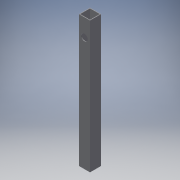
# Autodesk Inventor part: CounterWeight
Saved by Autodesk Inventor 2019.3 (Build 233278000, 278)
## iProperties
Created: 2019-07-02
Part Number: CounterWeight
Material: Generic
Document SubType Name: Modeling
Designer: mark
Density: 1 g/cm^3
Appearance: Default
Author: mark
Autodesk Inventor part; units mm, degrees
ref_plane "YZ Plane" through (0, 0, 0) normal (1, 0, 0) x (0, 1, 0)
ref_plane "XZ Plane" through (0, 0, 0) normal (0, 1, 0) x (-1, 0, 0)
ref_plane "XY Plane" through (0, 0, 0) normal (0, 0, 1) x (1, 0, 0)
sketch "Sketch1" plane through (0, 0, 0) normal (0, 0, 1) x (1, 0, 0)
  line L0 (0, 0) -> (25.4, 0) projected
  line L1 (25.4, 0) -> (25.4, 500) projected
  line L2 (0, 500) -> (25.4, 500) projected
  line L3 (0, 0) -> (0, 500) projected
  line L4 (23.8125, 0) -> (23.8125, 500) projected
  line L5 (1.5875, 0) -> (1.5875, 500) projected
  line L6 (25.4, 50) -> (0, 50)
  line L7 (0, 50) -> (0, -250)
  line L8 (0, -250) -> (25.4, -250)
  line L9 (25.4, -250) -> (25.4, 50)
  dimension "d0" = 50
  dimension "d1" = 300
  constraints: 8 end point, 2 collinear
  measures "d0" distance between parallel lines of L6 L0
  measures "d1" distance between parallel lines of L6 L8
extrude "Extrusion1" add sketch "Sketch1" along normal blind 25.4 contours L3 L6 L5 L0 | L0 L9 L8 L7 | L5 L6 L4 L0 | L4 L6 L1 L0
sketch "Sketch2" plane through (0, 50, 0) normal (0, 1, 0) x (1, 0, 0)
  line L0 (23.8125, -1.5875) -> (1.5875, -1.5875)
  line L1 (1.5875, -1.5875) -> (1.5875, -23.8125)
  line L2 (1.5875, -23.8125) -> (23.8125, -23.8125)
  line L3 (23.8125, -23.8125) -> (23.8125, -1.5875)
  line L4 (23.8125, 23.8125) -> (23.8125, 1.5875) projected
  line L5 (1.5875, 1.5875) -> (1.5875, 23.8125) projected
  line L6 (25.4, -25.4) -> (0, -25.4) projected
  point P0 (0, 0)
  dimension "d4" = 22.225
  dimension "d5" = 1.5875
  constraints: 8 end point, 2 collinear
  measures "d4" distance between parallel lines of L2 L0
  measures "d5" distance between parallel lines of L2 L6
extrude "Extrusion2" cut sketch "Sketch2" against normal up to next
sketch "Sketch3" plane through (0, 0, 25.4) normal (0, 0, 1) x (1, 0, 0)
  circle A0 centre (12.7, 10) radius 7.5
  line L0 (25.4, -250) -> (25.4, 50) projected
  line L1 (0, 0) -> (25.4, 0) projected
  line L2 (0, 0) -> (25.4, 0) projected
  line L3 (23.8125, 15.05) -> (1.5875, 15.05)
  dimension "d8" = 15
  dimension "d9" = 12.7
  dimension "d10" = 10
  constraints: 2 end point, 1 centre point, 1 horizontal, 2 other
  measures "d8" diameter of A0
  measures "d9" distance from line of L0 A0.centre
  measures "d10" distance from line of L1 A0.centre
extrude "Extrusion3" cut sketch "Sketch3" against normal up to next
sketch "Sketch4" plane through (1.5875, 50, 1.5875) normal (0, 0, 1) x (1, 0, 0)
  circle A0 centre (11.1125, -40) radius 7.5 projected
  circle A1 centre (11.1125, -40) radius 4.5
  point P0 (-1.5875, -50)
  dimension "d13" = 9
  constraints: 1 centre point, 1 coincident
  measures "d13" diameter of A1
extrude "Extrusion4" cut sketch "Sketch4" against normal up to next contours A1
body "Solid1"
